Autodesk Fusion 360 part; units mm, degrees
(part 3 of 3)
  spline S37 degree 5 poles (-31.8463, 21.6348) (-31.8387, 21.6182) (-31.8236, 21.585) (-31.8007, 21.5353) (-31.7701, 21.4693) (-31.7314, 21.387) (-31.6925, 21.3049) (-31.6532, 21.2232) (-31.6135, 21.1418) (-31.5736, 21.0606) (-31.5333, 20.9798) (-31.4926, 20.8992) (-31.4516, 20.8189) (-31.4103, 20.739) (-31.3687, 20.6594) (-31.3267, 20.58) (-31.2844, 20.501) (-31.2417, 20.4223) (-31.1987, 20.3439) (-31.1553, 20.2659) (-31.1116, 20.1882) (-31.0676, 20.1108) (-31.0232, 20.0337) (-30.9785, 19.957) (-30.9334, 19.8806) (-30.888, 19.8046) (-30.8422, 19.7289) (-30.796, 19.6536) (-30.7496, 19.5787) (-30.7027, 19.5041) (-30.6555, 19.4299) (-30.608, 19.356) (-30.5601, 19.2825) (-30.5118, 19.2094) (-30.4631, 19.1368) (-30.4141, 19.0645) (-30.3647, 18.9925) (-30.315, 18.921) (-30.2649, 18.85) (-30.2144, 18.7793) (-30.1635, 18.709) (-30.1123, 18.6392) (-30.0606, 18.5699) (-30.0086, 18.5009) (-29.9561, 18.4325) (-29.9033, 18.3645) (-29.8501, 18.297) (-29.7965, 18.2299) (-29.7425, 18.1633) (-29.6881, 18.0972) (-29.6333, 18.0316) (-29.578, 17.9666) (-29.5222, 17.9021) (-29.466, 17.8383) (-29.4094, 17.775) (-29.3523, 17.7122) (-29.2948, 17.65) (-29.2369, 17.5883) (-29.1786, 17.5272) (-29.1198, 17.4666) (-29.0604, 17.4069) (-29.0004, 17.348) (-28.9396, 17.2901) (-28.8782, 17.2332) (-28.8162, 17.1772) (-28.7537, 17.1217) (-28.6909, 17.0668) (-28.6278, 17.0123) (-28.5642, 16.9585) (-28.4998, 16.906) (-28.434, 16.8556) (-28.3799, 16.8175) (-28.3382, 16.7905) (-28.3099, 16.7732) (-28.2957, 16.7647) knots -1 -1 -1 -1 -1 -1 -0.98571429 -0.97142857 -0.95714286 -0.94285714 -0.92857143 -0.91428571 -0.9 -0.88571429 -0.87142857 -0.85714286 -0.84285714 -0.82857143 -0.81428571 -0.8 -0.78571429 -0.77142857 -0.75714286 -0.74285714 -0.72857143 -0.71428571 -0.7 -0.68571429 -0.67142857 -0.65714286 -0.64285714 -0.62857143 -0.61428571 -0.6 -0.58571429 -0.57142857 -0.55714286 -0.54285714 -0.52857143 -0.51428571 -0.5 -0.48571429 -0.47142857 -0.45714286 -0.44285714 -0.42857143 -0.41428571 -0.4 -0.38571429 -0.37142857 -0.35714286 -0.34285714 -0.32857143 -0.31428571 -0.3 -0.28571429 -0.27142857 -0.25714286 -0.24285714 -0.22857143 -0.21428571 -0.2 -0.18571429 -0.17142857 -0.15714286 -0.14285714 -0.12857143 -0.11428571 -0.1 -0.08571429 -0.07142857 -0.05714286 -0.04285714 -0.02857143 -0.01428571 0 0 0 0 0 0
  line L37 (-28.2957, 16.7647) -> (-27.7863, 16.4626)
  arc A75 (-27.1922, 14.356) -> (-27.7863, 16.4626) centre (-28.5961, 15.0972) ccw
  arc A76 (-27.1922, 14.356) -> (-27.5975, 13.5607) centre (0, 0) ccw
  arc A77 (-29.6509, 12.8031) -> (-27.5975, 13.5607) centre (-29.0223, 14.2608) ccw
  line L38 (-29.6509, 12.8031) -> (-30.1947, 13.0376)
  spline S38 degree 5 poles (-30.1947, 13.0376) (-30.21, 13.0442) (-30.2406, 13.0569) (-30.2869, 13.0748) (-30.3496, 13.0962) (-30.429, 13.1197) (-30.5094, 13.141) (-30.5903, 13.1608) (-30.6714, 13.1798) (-30.7528, 13.1984) (-30.8344, 13.2163) (-30.9162, 13.2335) (-30.9983, 13.2498) (-31.0808, 13.2649) (-31.1637, 13.2788) (-31.247, 13.2917) (-31.3305, 13.3037) (-31.4142, 13.315) (-31.4982, 13.3255) (-31.5823, 13.3355) (-31.6666, 13.3448) (-31.7511, 13.3534) (-31.8359, 13.3614) (-31.9208, 13.3686) (-32.0059, 13.3751) (-32.0911, 13.3809) (-32.1766, 13.3861) (-32.2622, 13.3906) (-32.348, 13.3946) (-32.4339, 13.3979) (-32.52, 13.4007) (-32.6062, 13.4029) (-32.6925, 13.4045) (-32.779, 13.4055) (-32.8656, 13.4059) (-32.9523, 13.4058) (-33.0392, 13.4051) (-33.1262, 13.4038) (-33.2132, 13.4021) (-33.3004, 13.3997) (-33.3877, 13.3969) (-33.4751, 13.3935) (-33.5626, 13.3896) (-33.6502, 13.3852) (-33.7379, 13.3803) (-33.8257, 13.3748) (-33.9136, 13.3689) (-34.0016, 13.3624) (-34.0896, 13.3555) (-34.1778, 13.348) (-34.266, 13.3401) (-34.3542, 13.3317) (-34.4426, 13.3228) (-34.531, 13.3134) (-34.6195, 13.3035) (-34.7081, 13.2932) (-34.7967, 13.2824) (-34.8854, 13.2711) (-34.9741, 13.2594) (-35.063, 13.2472) (-35.1518, 13.2345) (-35.2407, 13.2214) (-35.3297, 13.2078) (-35.4187, 13.1938) (-35.5078, 13.1793) (-35.5969, 13.1644) (-35.686, 13.1491) (-35.7752, 13.1333) (-35.8644, 13.117) (-35.9537, 13.1003) (-36.043, 13.0832) (-36.1145, 13.0692) (-36.1681, 13.0584) (-36.2038, 13.0512) (-36.2217, 13.0476) knots 0 0 0 0 0 0 0.01428571 0.02857143 0.04285714 0.05714286 0.07142857 0.08571429 0.1 0.11428571 0.12857143 0.14285714 0.15714286 0.17142857 0.18571429 0.2 0.21428571 0.22857143 0.24285714 0.25714286 0.27142857 0.28571429 0.3 0.31428571 0.32857143 0.34285714 0.35714286 0.37142857 0.38571429 0.4 0.41428571 0.42857143 0.44285714 0.45714286 0.47142857 0.48571429 0.5 0.51428571 0.52857143 0.54285714 0.55714286 0.57142857 0.58571429 0.6 0.61428571 0.62857143 0.64285714 0.65714286 0.67142857 0.68571429 0.7 0.71428571 0.72857143 0.74285714 0.75714286 0.77142857 0.78571429 0.8 0.81428571 0.82857143 0.84285714 0.85714286 0.87142857 0.88571429 0.9 0.91428571 0.92857143 0.94285714 0.95714286 0.97142857 0.98571429 1 1 1 1 1 1
  arc A78 (-36.2217, 13.0476) -> (-36.9731, 10.7349) centre (0, 0) ccw
  spline S39 degree 5 poles (-36.9731, 10.7349) (-36.9608, 10.7214) (-36.9361, 10.6946) (-36.8991, 10.6544) (-36.8495, 10.601) (-36.7873, 10.5347) (-36.7249, 10.4687) (-36.6623, 10.4031) (-36.5994, 10.3379) (-36.5363, 10.2731) (-36.473, 10.2086) (-36.4095, 10.1446) (-36.3457, 10.0809) (-36.2817, 10.0176) (-36.2175, 9.9548) (-36.153, 9.8923) (-36.0883, 9.8302) (-36.0235, 9.7686) (-35.9583, 9.7073) (-35.893, 9.6465) (-35.8274, 9.5861) (-35.7616, 9.5261) (-35.6956, 9.4665) (-35.6293, 9.4074) (-35.5629, 9.3487) (-35.4962, 9.2904) (-35.4292, 9.2326) (-35.3621, 9.1752) (-35.2947, 9.1183) (-35.2271, 9.0618) (-35.1593, 9.0058) (-35.0912, 8.9503) (-35.023, 8.8952) (-34.9545, 8.8406) (-34.8857, 8.7865) (-34.8168, 8.7329) (-34.7476, 8.6798) (-34.6782, 8.6271) (-34.6086, 8.575) (-34.5387, 8.5234) (-34.4686, 8.4723) (-34.3983, 8.4218) (-34.3277, 8.3717) (-34.257, 8.3223) (-34.1859, 8.2734) (-34.1147, 8.225) (-34.0432, 8.1773) (-33.9715, 8.13) (-33.8996, 8.0834) (-33.8274, 8.0373) (-33.755, 7.9919) (-33.6823, 7.9471) (-33.6094, 7.9031) (-33.5362, 7.8597) (-33.4627, 7.817) (-33.389, 7.775) (-33.3151, 7.7336) (-33.241, 7.6928) (-33.1666, 7.6526) (-33.092, 7.6133) (-33.0171, 7.5748) (-32.9418, 7.5373) (-32.8662, 7.5011) (-32.7902, 7.4659) (-32.7139, 7.4318) (-32.6373, 7.3983) (-32.5606, 7.3655) (-32.4838, 7.3332) (-32.4067, 7.3017) (-32.3292, 7.2716) (-32.251, 7.244) (-32.1878, 7.2245) (-32.1398, 7.2117) (-32.1076, 7.204) (-32.0914, 7.2004) knots -1 -1 -1 -1 -1 -1 -0.98571429 -0.97142857 -0.95714286 -0.94285714 -0.92857143 -0.91428571 -0.9 -0.88571429 -0.87142857 -0.85714286 -0.84285714 -0.82857143 -0.81428571 -0.8 -0.78571429 -0.77142857 -0.75714286 -0.74285714 -0.72857143 -0.71428571 -0.7 -0.68571429 -0.67142857 -0.65714286 -0.64285714 -0.62857143 -0.61428571 -0.6 -0.58571429 -0.57142857 -0.55714286 -0.54285714 -0.52857143 -0.51428571 -0.5 -0.48571429 -0.47142857 -0.45714286 -0.44285714 -0.42857143 -0.41428571 -0.4 -0.38571429 -0.37142857 -0.35714286 -0.34285714 -0.32857143 -0.31428571 -0.3 -0.28571429 -0.27142857 -0.25714286 -0.24285714 -0.22857143 -0.21428571 -0.2 -0.18571429 -0.17142857 -0.15714286 -0.14285714 -0.12857143 -0.11428571 -0.1 -0.08571429 -0.07142857 -0.05714286 -0.04285714 -0.02857143 -0.01428571 0 0 0 0 0 0
  line L39 (-32.0914, 7.2004) -> (-31.5136, 7.0705)
  arc A79 (-30.2976, 5.2505) -> (-31.5136, 7.0705) centre (-31.8618, 5.5216) ccw
  circle A80 centre (0, 0) radius 7.5
  dimension "d9" = 15
  constraint coincident A0.centre A2.centre
  measures "d9" diameter of A80
extrude "Extruir3" add sketch "Boceto2 (2)" along normal blind 50 contours A80 bodies 1 in component "Spur Gear (20 teeth)"
sketch "Boceto3 (2)" plane through (0, 0, 63) normal (0, 0, 1) x (-1, 0, 0)
  circle A0 centre (0, 0) radius 7.5
  circle A1 centre (0, 0) radius 7.5
  constraint coincident A0.centre A1.centre
extrude "Extruir4" add sketch "Boceto3 (2)" along normal blind 15.297 bodies 1 in component "Spur Gear (20 teeth)"
sketch "Boceto4" plane through (0, 0, 78.297) normal (0, 0, 1) x (-1, 0, 0)
  circle A0 centre (0, 0) radius 7.5
  circle A1 centre (0, 0) radius 15
  dimension "d14" = 30
  constraint concentric A0 A1
  measures "d14" diameter of A1
extrude "Extruir1'" add sketch "Boceto4" along normal blind 2 separate body makes body 2
sketch "Boceto5" plane through (0, 0, 78.297) normal (0, 0, 1) x (-1, 0, 0)
  circle A0 centre (0, 0) radius 7.5
  circle A1 centre (0, 0) radius 7.5
  constraint coincident A0.centre A1.centre
extrude "Extruir2'" add sketch "Boceto5" along normal blind 2 bodies 2
sketch "Boceto6" plane through (0, 0, 80.297) normal (0, 0, 1) x (-1, 0, 0)
  circle A0 centre (0, 0) radius 15
  circle A1 centre (0, 12) radius 1
  circle A2 centre (-12, 0) radius 1
  circle A3 centre (12, 0) radius 1
  circle A4 centre (0, -12) radius 1
  dimension "d19" = 12
  dimension "d20" = 12
  dimension "d21" = 12
  dimension "d22" = 12
  dimension "d23" = 2
  dimension "d24" = 2
  dimension "d25" = 2
  dimension "d26" = 2
  measures "d19" distance of A0.centre A1.centre
  measures "d20" distance of A0.centre A2.centre
  measures "d21" distance of A0.centre A4.centre
  measures "d22" distance of A0.centre A3.centre
  measures "d23" diameter of A1
  measures "d24" diameter of A2
  measures "d25" diameter of A4
  measures "d26" diameter of A3
extrude "Extruir3'" cut sketch "Boceto6" against normal blind 2 contours A1 | A2 | A3 | A4 bodies 2
component "Spur Gear (20 teeth)" placed x (1, 0, 0) y (0, 1, 0) z (0, 0, 1) at (0, 0, 0)
